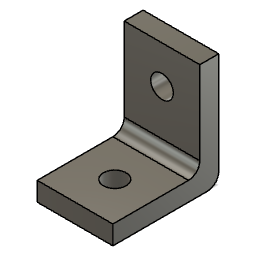
Double Door Opener 3 v7 (Autodesk Fusion 360 design; units mm, degrees)
Autodesk Fusion 360 part; units mm, degrees
sketch "Sketch1" plane through (0, 0, 0) normal (0, 1, 0) x (1, 0, 0)
  line L0 (5, 6.5) -> (-5, 6.5)
  line L1 (-5, 6.5) -> (-5, -6.5)
  line L2 (-5, -6.5) -> (5, -6.5)
  line L3 (5, -6.5) -> (5, 6.5)
  line L4 (5, 6.5) -> (-5, -6.5) construction
  line L5 (-5, 6.5) -> (5, -6.5) construction
  circle A0 centre (0, -1.25) radius 1.5
  dimension "d1" = 13
  dimension "d2" = 10
  dimension "d21" = 3
  dimension "d22" = 1.25
  constraint horizontal L0
  constraint perpendicular L0 L1
  constraint parallel L0 L2
  constraint parallel L1 L3
  constraint coincident L4 origin
  constraint coincident L5 origin
  measures "d1" distance of L0.end L1.end
  measures "d2" distance of L0.start L0.end
  measures "d21" diameter of A0
  measures "d22" distance of origin A0.centre
extrude "Extrude1" add sketch "Sketch1" along normal blind 2.5
sketch "Sketch3" plane through (0, 0, 0) normal (0, 1, 0) x (1, 0, 0)
  line L0 (-5, 5) -> (5, 5)
  line L1 (5, 5) -> (5, 7.5)
  line L2 (5, 7.5) -> (-5, 7.5)
  line L3 (-5, 7.5) -> (-5, 5)
  dimension "d10" = 2.5
  dimension "d11" = 10
  dimension "d12" = 5
  dimension "d13" = 5
  constraint horizontal L0
  constraint vertical L1
  constraint horizontal L2
  constraint vertical L3
  measures "d10" distance of L0.start L2.end
  measures "d11" distance of L1.end L2.end
  measures "d12" vertical distance of origin L0.end
  measures "d13" horizontal distance of origin L0.start
extrude "Extrude3" add sketch "Sketch3" along normal blind 15
sketch "Sketch5" plane through (0, 0, -5) normal (0, 0, 1) x (1, 0, 0)
  line L0 (5, 2.5) -> (5, 15)
  line L1 (5, 15) -> (-5, 15)
  line L2 (-5, 15) -> (-5, 2.5)
  circle A0 centre (0, 10) radius 1.5
  line L3 (-5, 2.5) -> (5, 2.5)
  dimension "d16" = 5
  dimension "d17" = 3
  constraint vertical origin A0.centre
  measures "d16" vertical distance of L1.end A0.centre
  measures "d17" diameter of A0
extrude "Extrude4" cut sketch "Sketch5" against normal blind 45 contours A0
fillet "Fillet1" radius 1.5 2 edges at (0, 2.5, -5) (0, 0, -7.5)
